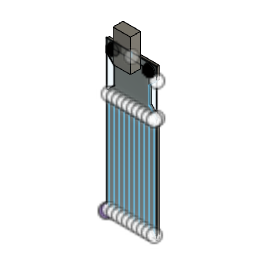
Aquapella (Autodesk Fusion 360 archive; units mm, degrees)
design "Water Sensor"
Autodesk Fusion 360 part; units mm, degrees
sketch "Sketch1" plane through (0, 0, 0) normal (0, 1, 0) x (1, 0, 0)
  line L0 (0, 0) -> (20, 0)
  line L1 (20, 0) -> (20, -60)
  line L2 (20, -60) -> (0, -60)
  line L3 (0, -60) -> (0, 0)
  circle A0 centre (2.75, -57.5) radius 2
  line L4 (2.75, -60) -> (17.25, -60)
  line L5 (17.25, -60) -> (17.25, -57.5)
  line L6 (17.25, -57.5) -> (2.75, -57.5)
  circle A1 centre (17.25, -57.5) radius 2
  line L7 (0, -60) -> (0, -55)
  line L8 (10, -60) -> (10, -58.5)
  line L9 (3, -52) -> (3, -45)
  line L10 (0, -55) -> (3, -52)
  line L11 (3, -45) -> (0, -42)
  line L12 (20, -55) -> (17, -52)
  line L13 (17, -52) -> (17, -45)
  line L14 (17, -45) -> (20, -42)
  line L15 (1, -1) -> (1, -41)
  line L16 (3, -1) -> (3, -41)
  line L17 (5, -1) -> (5, -41)
  line L18 (7, -1) -> (7, -41)
  line L19 (9, -1) -> (9, -41)
  line L20 (11, -1) -> (11, -41)
  line L21 (13, -1) -> (13, -41)
  line L22 (15, -1) -> (15, -41)
  line L23 (17, -1) -> (17, -41)
  line L24 (19, -1) -> (19, -41)
  line L25 (2.75, -60) -> (2.75, -57.5)
  dimension "d1" = 60
  dimension "d2" = 20
  dimension "d20" = 3
  dimension "d21" = 8
  dimension "d22" = 18
  dimension "d23" = 7
  dimension "d24" = 5
  dimension "d27" = 18
  dimension "d28" = 0
  dimension "d29" = 2.5
  dimension "d30" = 2.75
  dimension "d31" = 14.5
  dimension "d32" = 2.75
  dimension "d33" = 4
  dimension "d34" = 4
  constraint horizontal L0
  constraint vertical L1
  constraint horizontal L2
  constraint vertical L3
  constraint coincident L0.start L3.end
  constraint horizontal L4
  constraint vertical L5
  constraint coincident L2 L4.start
  constraint coincident L5.end L6.start
  constraint midpoint L2 L8.start
  constraint parallel L3 L9
  constraint coincident L3 L11.end
  constraint collinear L3 L7
  constraint symmetric L8 L7.end L12.start
  constraint symmetric L8 L9.start L12.end
  constraint symmetric L8 L9.end L13.end
  constraint symmetric L8 L11.end L14.end
  constraint perpendicular L0 L15
  constraint perpendicular L5 L6
  constraint perpendicular L6 L25
  constraint coincident A0.centre L6.end
  measures "d1" distance of L0.start L2.end
  measures "d2" distance of L1 L3
  measures "d20" distance of L3 L9
  measures "d21" distance of L2 L9.start
  measures "d22" distance of L2 L11.end
  measures "d23" distance of L9.start L9.end
  measures "d24" distance of L2.end L7.end
  measures "d29" distance of L2 L6
  measures "d30" distance of L3 L25
  measures "d31" distance of L5 L25
  measures "d32" distance of L1 L5
  measures "d33" diameter of A0
  measures "d34" diameter of A1
extrude "Extrude1" add sketch "Sketch1" along normal blind 1 contours L0 L1 L2 L3 A0 L5 L6 A1 L7 L9 L10 L11 L12 L13 L14 L25 | L2 A0 L4 L5 L6 A1 L25
sketch "Sketch2" plane through (0, 0, 0) normal (0, -1, 0) x (1, 0, 0)
  circle A0 centre (2.75, 57.5) radius 2
  circle A1 centre (17.25, 57.5) radius 2
  line L0 (20, 60) -> (0, 60)
  line L1 (0, 42) -> (0, 0)
  line L2 (0, 0) -> (20, 0)
  line L3 (20, 0) -> (20, 42)
  line L4 (6.5, 59) -> (13.5, 59)
  line L5 (13.5, 59) -> (13.5, 56)
  line L6 (13.5, 56) -> (6.5, 56)
  line L7 (6.5, 56) -> (6.5, 59)
  line L8 (10, 60) -> (10, 59)
  line L9 (17, 52) -> (20, 55)
  line L10 (20, 55) -> (20, 60)
  line L11 (0, 60) -> (0, 55)
  line L12 (0, 55) -> (3, 52)
  line L13 (3, 52) -> (3, 45)
  line L14 (3, 45) -> (0, 42)
  line L15 (20, 42) -> (17, 45)
  line L16 (17, 45) -> (17, 52)
  dimension "d13" = 1
  dimension "d14" = 7
  dimension "d15" = 3
  constraint horizontal L4
  constraint vertical L5
  constraint horizontal L6
  constraint vertical L7
  constraint midpoint L0 L8.start
  constraint coincident L4 L8.end
  constraint perpendicular L4 L8
  constraint midpoint L4 L8.end
  measures "d13" distance of L0 L4
  measures "d14" distance of L5 L7
  measures "d15" distance of L4 L6
extrude "Extrude2" add sketch "Sketch2" along normal blind 4 contours L4 L5 L6 L7
extrude "Extrude3" add 1 faces at (8.8333, -2.6667, 59) along direction (0, 0, 1) blind 10

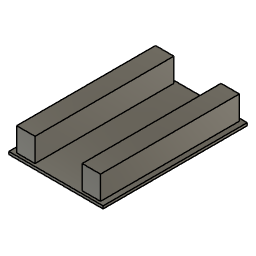
design "Ardunio Mount"
Autodesk Fusion 360 part; units mm, degrees
sketch "Sketch1" plane through (0, 0, 0) normal (0, 0, 1) x (1, 0, 0)
  line L0 (0, 0) -> (36, 0)
  line L1 (36, 0) -> (36, 55)
  line L2 (36, 55) -> (0, 55)
  line L3 (0, 55) -> (0, 0)
  dimension "d1" = 36
  dimension "d2" = 55
  constraint horizontal L0
  constraint vertical L1
  constraint horizontal L2
  constraint vertical L3
  constraint coincident L0.start L3.end
  measures "d1" distance of L0.start L0.end
  measures "d2" distance of L0.start L2.end
extrude "Extrude1" add sketch "Sketch1" along normal blind 1
sketch "Sketch3" plane through (0, 0, 1) normal (0, 0, 1) x (-1, 0, 0)
  line L0 (0, -55) -> (0, 0)
  line L1 (0, 0) -> (-36, 0)
  line L2 (-36, 0) -> (-36, -55)
  line L3 (-36, -55) -> (0, -55)
  line L4 (-2, -1) -> (-9, -1)
  line L5 (-9, -1) -> (-9, -54)
  line L6 (-9, -54) -> (-2, -54)
  line L7 (-2, -54) -> (-2, -1)
  line L8 (-18, -55) -> (-18, 0)
  line L9 (-27, -1) -> (-27, -54)
  line L10 (-27, -54) -> (-34, -54)
  line L11 (-34, -54) -> (-34, -1)
  line L12 (-34, -1) -> (-27, -1)
  dimension "d5" = 2
  dimension "d6" = 1
  dimension "d7" = 7
  dimension "d8" = 1
  constraint horizontal L4
  constraint vertical L5
  constraint horizontal L6
  constraint vertical L7
  constraint midpoint L3 L8.start
  constraint midpoint L1 L8.end
  constraint symmetric L4.start L8 L11.end
  constraint symmetric L4.end L8 L9.start
  constraint symmetric L5.end L8 L9.end
  constraint symmetric L6.end L8 L10.end
  measures "d5" distance of L0 L7
  measures "d6" distance of L1 L4
  measures "d7" distance of L5 L7
  measures "d8" distance of L3 L6
extrude "Extrude2" add sketch "Sketch3" along normal blind 9 contours L4 L5 L6 L7 | L9 L10 L11 L12
sketch "Sketch4" plane through (0, 0, 0) normal (0, 0, -1) x (1, 0, 0)
  line L0 (0, 0) -> (0, -55)
  line L1 (0, -55) -> (36, -55)
  line L2 (36, -55) -> (36, 0)
  line L3 (36, 0) -> (0, 0)
  circle A0 centre (5, -3) radius 0.25
  circle A1 centre (31, -3) radius 0.25
  circle A2 centre (5, -6.7692) radius 0.25
  circle A3 centre (31, -6.7692) radius 0.25
  circle A4 centre (5, -10.5385) radius 0.25
  circle A5 centre (31, -10.5385) radius 0.25
  circle A6 centre (5, -14.3077) radius 0.25
  circle A7 centre (31, -14.3077) radius 0.25
  circle A8 centre (5, -18.0769) radius 0.25
  circle A9 centre (31, -18.0769) radius 0.25
  circle A10 centre (5, -21.8462) radius 0.25
  circle A11 centre (31, -21.8462) radius 0.25
  circle A12 centre (5, -25.6154) radius 0.25
  circle A13 centre (31, -25.6154) radius 0.25
  circle A14 centre (5, -29.3846) radius 0.25
  circle A15 centre (31, -29.3846) radius 0.25
  circle A16 centre (5, -33.1538) radius 0.25
  circle A17 centre (31, -33.1538) radius 0.25
  circle A18 centre (5, -36.9231) radius 0.25
  circle A19 centre (31, -36.9231) radius 0.25
  circle A20 centre (5, -40.6923) radius 0.25
  circle A21 centre (31, -40.6923) radius 0.25
  circle A22 centre (5, -44.4615) radius 0.25
  circle A23 centre (31, -44.4615) radius 0.25
  circle A24 centre (5, -48.2308) radius 0.25
  circle A25 centre (31, -48.2308) radius 0.25
  circle A26 centre (5, -52) radius 0.25
  circle A27 centre (31, -52) radius 0.25
  dimension "d11" = 0.5
  dimension "d12" = 5
  dimension "d13" = 3
  dimension "d16" = 26
  dimension "d17" = -49
  measures "d11" diameter of A0
  measures "d12" distance of L0 A0.centre
  measures "d13" distance of L3 A0.centre
extrude "Extrude3" add sketch "Sketch4" along normal blind 2 contours A0 | A1 | A2 | A3 | A4 | A5 | A6 | A7 | A8 | A9 | A10 | A11 | A12 | A13 | A14 | A15 | A16 | A17 | A18 | A19 | A20 | A21 | A22 | A23 | A24 | A25 | A26 | A27
